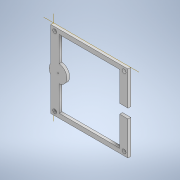
# Autodesk Inventor part: P4
Saved by Autodesk Inventor 2022 (Build 260153000, 153)
## iProperties
Created: 2022-11-21
Part Number: P4
Material: Genérico
Document SubType Name: Modeling
Designer: javie
Density: 1 g/cm^3
Appearance: Valor por defecto
Author: javie
Autodesk Inventor part; units mm, degrees
ref_plane "YZ Plane" through (0, 0, 0) normal (1, 0, 0) x (0, 1, 0)
ref_plane "XZ Plane" through (0, 0, 0) normal (0, 1, 0) x (-1, 0, 0)
ref_plane "XY Plane" through (0, 0, 0) normal (0, 0, 1) x (1, 0, 0)
sketch "Boceto1" plane through (0, 0, 0) normal (0, 0, 1) x (1, 0, 0)
  circle A0 centre (7, -7) radius 3.5
  circle A1 centre (133, -7) radius 3.5
  circle A2 centre (7, -133) radius 3.5
  circle A3 centre (133, -133) radius 3.5
  line L0 (125, -117.6199) -> (125, -132)
  line L1 (125, -132) -> (15, -132)
  line L2 (15, -132) -> (15, -118)
  line L3 (15, -118) -> (15, -85.8745)
  arc A4 (0, -60.6726) -> (0, -79.3274) centre (13, -70) ccw
  line L4 (15, -54.1255) -> (15, -8)
  line L5 (15, -8) -> (125, -8)
  line L6 (125, -8) -> (125, -61.5)
  line L7 (125, -61.5) -> (140, -61.5)
  line L8 (140, -61.5) -> (140, 0)
  line L9 (140, 0) -> (0, 0)
  line L10 (0, 0) -> (0, -60.6726)
  line L11 (0, -79.3274) -> (0, -140)
  line L12 (0, -140) -> (140, -140)
  line L13 (140, -140) -> (140, -78.5)
  line L14 (140, -78.5) -> (125, -78.5)
  line L15 (125, -78.5) -> (125, -118)
  arc A5 (15, -85.8745) -> (15, -54.1255) centre (13, -70) ccw
  circle A6 centre (13, -70) radius 1
  point P0 (15, -54.1255)
  point P1 (0, -60.6726)
  point P2 (0, -79.3274)
  dimension "d0" = 2
  constraints: 32 end point, 7 centre point, 4 point on circle, 1 coincident
  measures "d0" diameter of A6
extrude "Extrusión1" add sketch "Boceto1" along normal blind 5
